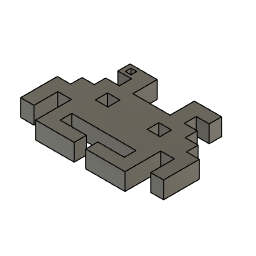
keychain_v2 (Autodesk Fusion 360 design; units mm, degrees)
Autodesk Fusion 360 part; units mm, degrees
note: some values were not read from the file. Set by a fixed rule: which face or edge a step refers to.
sketch "measurements" plane through (0, 0, 0) normal (0, 0, 1) x (1, 0, 0)
  line L0 (-76.9792, 43.6447, -4.0233) -> (23.0208, 43.6447, -4.0233)
  line L1 (23.0208, 43.6447, -4.0233) -> (23.0208, -26.3553, -4.0233)
  line L2 (23.0208, -26.3553, -4.0233) -> (-76.9792, -26.3553, -4.0233)
  line L3 (-76.9792, -26.3553, -4.0233) -> (-76.9792, 43.6447, -4.0233)
  dimension "d1" = 100
  dimension "d2" = 70
sketch "body" plane through (0, 0, 0) normal (0, 0, 1) x (1, 0, 0)
  line L0 (-77.8145, -17.6466) -> (-68.4918, -17.6466)
  line L1 (-68.4918, -17.6466) -> (-68.4918, -1)
  line L2 (-68.4918, -1) -> (-59, -1)
  line L3 (-59, -1) -> (-59, -17.6466)
  line L4 (-59, -17.6466) -> (-59, -26)
  line L5 (-59, -26) -> (-32, -26)
  line L6 (-32, -26) -> (-32, -17.4454)
  line L7 (-32, -17.4454) -> (-50.398, -17.4454)
  line L8 (-50.398, -17.4454) -> (-50.398, -9.3233)
  line L9 (-50.398, -9.3233) -> (-5.4815, -9.3233)
  line L10 (-5.4815, -9.3233) -> (-5.4815, -17.492)
  line L11 (-5.4815, -17.492) -> (-24, -17.492)
  line L12 (-24, -17.492) -> (-24, -26)
  line L13 (-24, -26) -> (3.4738, -26)
  line L14 (3.4738, -26) -> (3.4738, -1)
  line L15 (3.4738, -1) -> (13, -1)
  line L16 (13, -1) -> (13, -17.5434)
  line L17 (13, -17.5434) -> (22, -17.5434)
  line L18 (22, -17.5434) -> (22, 7.5189)
  line L19 (22, 7.5189) -> (13, 7.5189)
  line L20 (13, 7.5189) -> (13, 15.6438)
  line L21 (13, 15.6438) -> (4, 15.6438)
  line L22 (4, 15.6438) -> (4, 24)
  line L23 (4, 24) -> (-5, 24)
  line L24 (-5, 24) -> (-5, 32.3456)
  line L25 (-5, 32.3456) -> (4, 32.3456)
  line L26 (4, 32.3456) -> (4, 41)
  line L27 (4, 41) -> (-15, 41)
  line L28 (-15, 41) -> (-15, 24)
  line L29 (-15, 24) -> (-41, 24)
  line L30 (-41, 24) -> (-41, 41)
  line L31 (-41, 41) -> (-60, 41)
  line L32 (-60, 41) -> (-60, 32.5)
  line L33 (-60, 32.5) -> (-50.5, 32.5)
  line L34 (-50.5, 32.5) -> (-50.5, 24)
  line L35 (-50.5, 24) -> (-60, 24)
  line L36 (-60, 24) -> (-60, 16)
  line L37 (-60, 16) -> (-68.5245, 16)
  line L38 (-68.5245, 16) -> (-68.5245, 8)
  line L39 (-68.5245, 8) -> (-77.8145, 8)
  line L40 (-77.8145, 8) -> (-77.8145, -17.6466)
  line L41 (-50.2879, 15.5655) -> (-50.2879, 7.1611)
  line L42 (-50.2879, 7.1611) -> (-41.6942, 7.1611)
  line L43 (-41.6942, 7.1611) -> (-41.6942, 15.5655)
  line L44 (-41.6942, 15.5655) -> (-50.2879, 15.5655)
  line L45 (-14.3571, 15.4858) -> (-14.3571, 7.4265)
  line L46 (-14.3571, 7.4265) -> (-5.5085, 7.4265)
  line L47 (-5.5085, 7.4265) -> (-5.5085, 15.4858)
  line L48 (-5.5085, 15.4858) -> (-14.3571, 15.4858)
  line L49 (-57.073, 38.7445) -> (-53.073, 38.7445)
  line L50 (-53.073, 38.7445) -> (-53.073, 34.7445)
  line L51 (-53.073, 34.7445) -> (-57.073, 34.7445)
  line L52 (-57.073, 34.7445) -> (-57.073, 38.7445)
  dimension "d18" = 4
  dimension "d19" = 4
  constraint horizontal L0
  constraint perpendicular L0 L1
  constraint perpendicular L1 L2
  constraint perpendicular L2 L3
  constraint perpendicular L2 L4
  constraint perpendicular L3 L5
  constraint perpendicular L5 L6
  constraint perpendicular L6 L7
  constraint perpendicular L5 L8
  constraint perpendicular L8 L9
  constraint perpendicular L9 L10
  constraint perpendicular L6 L11
  constraint perpendicular L11 L12
  constraint perpendicular L12 L13
  constraint perpendicular L13 L14
  constraint perpendicular L14 L15
  constraint perpendicular L15 L16
  constraint perpendicular L16 L17
  constraint perpendicular L17 L18
  constraint perpendicular L18 L19
  constraint perpendicular L19 L20
  constraint perpendicular L20 L21
  constraint perpendicular L21 L22
  constraint perpendicular L22 L23
  constraint perpendicular L21 L24
  constraint perpendicular L24 L25
  constraint perpendicular L25 L26
  constraint perpendicular L26 L27
  constraint perpendicular L27 L28
  constraint perpendicular L28 L29
  constraint perpendicular L29 L30
  constraint perpendicular L28 L31
  constraint perpendicular L31 L32
  constraint perpendicular L28 L33
  constraint perpendicular L33 L34
  constraint perpendicular L34 L35
  constraint perpendicular L35 L36
  constraint perpendicular L36 L37
  constraint perpendicular L35 L38
  constraint perpendicular L38 L39
  constraint perpendicular L39 L40
  constraint vertical L41
  constraint perpendicular L41 L42
  constraint perpendicular L42 L43
  constraint perpendicular L41 L44
  constraint vertical L45
  constraint perpendicular L45 L46
  constraint perpendicular L46 L47
  constraint perpendicular L45 L48
  constraint horizontal L49
  constraint vertical L50
  constraint horizontal L51
  constraint vertical L52
  measures "d18" distance of L49.start L49.end
  measures "d19" distance of L49.end L50.end
sketch "Sketch3" plane through (0, 0, 0) normal (0, 0, 1) x (1, 0, 0)
extrude "Extrude1" add sketch "body" along normal blind 2 makes body 1
extrude "Extrude2" add 1 faces at (-32.5246, -3.8285, 0) along direction (0, 0, -1) blind 10 on bodies 1 bodies 1
copy_body "CopyPasteBodies1" bodies 1 makes body 2
move_body "Move1" bodies 2 to x (1, 0, 0) y (0, 1, 0) z (0, 0, 1) at (-148.467, -33.1463, 0)
shell "Shell1" thickness 1 outward yes removed faces 1 at (-180.9915, -36.9748, -10) on bodies 2
move_body "Move2" bodies 1 to x (1, 0, 0) y (0, 1, 0) z (0, 0, 1) at (-145.0599, -6.038, 8.6645)
move_body "Move3" bodies 2 to x (1, 0, 0) y (0, 1, 0) z (0, 0, 1) at (92.7922, -9.2176, 23.1215)
delete_face "DeleteFace2" 6 faces at (-64.4661, -27.8781, 21.7881) (-64.4661, -34.604, 13.1215) (-67.0822, -34.9373, 21.1215) (-61.1832, -32.2509, 21.1215) (-64.1327, -26.8781, 21.1215) (-70.0318, -29.5645, 21.1215) on bodies 2
delete_face "DeleteFace3" 5 faces at (-102.7647, -34.2028, 21.7881) (-100.2335, -26.7984, 17.1215) (-97.3689, -32.4013, 17.1215) (-103.0981, -35.2028, 17.1215) (-105.9626, -32.4013, 21.1215) on bodies 2
move_body "Move4" bodies 1 to x (1, 0, 0) y (0, 1, 0) z (0, 0, 1) at (89.1878, -35.4331, -0.5344)
move_body "Move5" bodies 1 to x (1, 0, 0) y (0, 1, 0) z (0, 0, 1) at (0, -183, 0)
scale "Scale1" factor 0.735339 about (-60.8721, -200.4711, -1.87) bodies 1
move_body "Move6" bodies 1 to x (1, 0, 0) y (0, 1, 0) z (0, 0, 1) at (-27.947, 35.9807, -65.7044)
move_body "Move7" bodies 1 to x (1, 0, 0) y (0, 1, 0) z (0, 0, 1) at (5.4665, 41.4487, -39.2545)
move_body "Move8" bodies 1 to x (1, 0, 0) y (0, 1, 0) z (0, 0, 1) at (5.1111, -23.3317, 85.8727)
move_body "Move9" bodies 1 to x (1, 0, 0) y (0, 1, 0) z (0, 0, 1) at (-3.4244, 72.2145, 50.5394)
move_body "Move10" bodies 1 to x (1, 0, 0) y (0, 1, 0) z (0, 0, 1) at (0, 65, 0)
move_body "Move11" bodies 1 to x (1, 0, 0) y (0, 1, 0) z (0, 0, 1) at (10, 20, 0)
move_body "Move12" bodies 1 to x (1, 0, 0) y (0, 1, 0) z (0, 0, 1) at (141.197, -29.9365, -10.1451)
sketch "Sketch4" plane through (0, 0, 25.1215) normal (0, 0, -1) x (1, 0, 0)
  line L0 (-133.4892, 60.0104) -> (-133.4892, 34.3638)
  line L1 (-133.4892, 34.3638) -> (-124.1992, 34.3638)
  line L2 (-124.1992, 34.3638) -> (-124.1992, 26.3638)
  line L3 (-124.1992, 26.3638) -> (-115.6747, 26.3638)
  line L4 (-115.6747, 26.3638) -> (-115.6747, 18.3638)
  line L5 (-115.6747, 18.3638) -> (-106.1747, 18.3638)
  line L6 (-106.1747, 18.3638) -> (-106.1747, 9.8638)
  line L7 (-106.1747, 9.8638) -> (-115.6747, 9.8638)
  line L8 (-115.6747, 9.8638) -> (-115.6747, 1.3638)
  line L9 (-115.6747, 1.3638) -> (-96.6747, 1.3638)
  line L10 (-96.6747, 1.3638) -> (-96.6747, 18.3638)
  line L11 (-96.6747, 18.3638) -> (-70.6747, 18.3638)
  line L12 (-70.6747, 18.3638) -> (-70.6747, 1.3638)
  line L13 (-70.6747, 1.3638) -> (-51.6747, 1.3638)
  line L14 (-51.6747, 1.3638) -> (-51.6747, 10.0183)
  line L15 (-51.6747, 10.0183) -> (-60.6747, 10.0183)
  line L16 (-60.6747, 10.0183) -> (-60.6747, 18.3638)
  line L17 (-60.6747, 18.3638) -> (-51.6747, 18.3638)
  line L18 (-51.6747, 18.3638) -> (-51.6747, 26.72)
  line L19 (-51.6747, 26.72) -> (-42.6747, 26.72)
  line L20 (-42.6747, 26.72) -> (-42.6747, 34.845)
  line L21 (-42.6747, 34.845) -> (-33.6747, 34.845)
  line L22 (-33.6747, 34.845) -> (-33.6747, 59.9073)
  line L23 (-33.6747, 59.9073) -> (-42.6747, 59.9073)
  line L24 (-42.6747, 59.9073) -> (-42.6747, 43.3638)
  line L25 (-42.6747, 43.3638) -> (-52.2009, 43.3638)
  line L26 (-52.2009, 43.3638) -> (-52.2009, 68.3638)
  line L27 (-52.2009, 68.3638) -> (-79.6747, 68.3638)
  line L28 (-79.6747, 68.3638) -> (-79.6747, 59.8559)
  line L29 (-79.6747, 59.8559) -> (-61.1562, 59.8559)
  line L30 (-61.1562, 59.8559) -> (-61.1562, 51.6871)
  line L31 (-61.1562, 51.6871) -> (-106.0727, 51.6871)
  line L32 (-106.0727, 51.6871) -> (-106.0727, 59.8092)
  line L33 (-106.0727, 59.8092) -> (-87.6747, 59.8092)
  line L34 (-87.6747, 59.8092) -> (-87.6747, 68.3638)
  line L35 (-87.6747, 68.3638) -> (-114.6747, 68.3638)
  line L36 (-114.6747, 68.3638) -> (-114.6747, 43.3638)
  line L37 (-114.6747, 43.3638) -> (-124.1665, 43.3638)
  line L38 (-124.1665, 43.3638) -> (-124.1665, 60.0104)
  line L39 (-124.1665, 60.0104) -> (-133.4892, 60.0104)
  line L40 (-112.7477, 7.6194) -> (-108.7477, 7.6194)
  line L41 (-108.7477, 7.6194) -> (-108.7477, 3.6194)
  line L42 (-108.7477, 3.6194) -> (-112.7477, 3.6194)
  line L43 (-112.7477, 3.6194) -> (-112.7477, 7.6194)
move_body "Move13" bodies 2 to x (1, 0, 0) y (0, 1, 0) z (0, 0, 1) at (5, 0, 0)
move_body "Move14" bodies 2 to x (-1, 0, 0) y (0, 1, 0) z (0, 0, -1) at (-229.3494, 0, 50.243)
move_body "Move15" bodies 1 to x (1, 0, 0) y (0, 1, 0) z (0, 0, 1) at (-26.9496, 1.9319, -5.2475)
torus "TorusPrimitive1" add centre line diameter 10 section diameter 5 placed x (1, 0, 0) y (0, 1, 0) z (0, 0, 1) at (16.8316, 16.8977, 0) separate body makes body 3
move_body "Move16" bodies 3 to x (1, 0, 0) y (0, 1, 0) z (0, 0, 1) at (-6.9234, -22.2268, 3.0483)
move_body "Move17" bodies 3 to x (1, 0, 0) y (0, 1, 0) z (0, 0, 1) at (0, 0, 10)
delete_face "DeleteFace4" 1 faces at (17.3494, -5.7005, 13.5437) on bodies 3
hidden bodies 2
named bodies: "key chain", "main base", "base)"
